Autodesk Fusion 360 part; units mm, degrees
(part 21 of 21)
  spline S194 degree 5 poles (-22.8173, 2.8931) (-22.8112, 2.8891) (-22.799, 2.8811) (-22.7807, 2.8692) (-22.7562, 2.8533) (-22.7256, 2.8337) (-22.695, 2.8142) (-22.6643, 2.7948) (-22.6336, 2.7755) (-22.6028, 2.7564) (-22.572, 2.7374) (-22.5411, 2.7186) (-22.5102, 2.6999) (-22.4793, 2.6814) (-22.4483, 2.6629) (-22.4173, 2.6447) (-22.3863, 2.6265) (-22.3552, 2.6085) (-22.3241, 2.5907) (-22.2929, 2.573) (-22.2617, 2.5554) (-22.2305, 2.538) (-22.1992, 2.5208) (-22.1679, 2.5037) (-22.1365, 2.4867) (-22.1051, 2.4699) (-22.0737, 2.4533) (-22.0422, 2.4368) (-22.0107, 2.4205) (-21.9792, 2.4043) (-21.9476, 2.3883) (-21.9159, 2.3724) (-21.8843, 2.3567) (-21.8526, 2.3412) (-21.8209, 2.3259) (-21.7891, 2.3107) (-21.7573, 2.2957) (-21.7254, 2.2808) (-21.6935, 2.2661) (-21.6616, 2.2517) (-21.6296, 2.2373) (-21.5976, 2.2232) (-21.5656, 2.2093) (-21.5335, 2.1955) (-21.5014, 2.1819) (-21.4693, 2.1686) (-21.4371, 2.1554) (-21.4048, 2.1424) (-21.3726, 2.1296) (-21.3403, 2.1171) (-21.3079, 2.1047) (-21.2755, 2.0926) (-21.2431, 2.0807) (-21.2107, 2.069) (-21.1782, 2.0575) (-21.1456, 2.0462) (-21.113, 2.0352) (-21.0804, 2.0245) (-21.0478, 2.0141) (-21.0151, 2.0039) (-20.9823, 1.9939) (-20.9495, 1.9842) (-20.9167, 1.9748) (-20.8838, 1.9657) (-20.8509, 1.9569) (-20.8179, 1.9485) (-20.7906, 1.9419) (-20.7698, 1.9371) (-20.7556, 1.9339) (-20.748, 1.9323) (-20.7471, 1.9321) knots -1 -1 -1 -1 -1 -1 -0.98571429 -0.97142857 -0.95714286 -0.94285714 -0.92857143 -0.91428571 -0.9 -0.88571429 -0.87142857 -0.85714286 -0.84285714 -0.82857143 -0.81428571 -0.8 -0.78571429 -0.77142857 -0.75714286 -0.74285714 -0.72857143 -0.71428571 -0.7 -0.68571429 -0.67142857 -0.65714286 -0.64285714 -0.62857143 -0.61428571 -0.6 -0.58571429 -0.57142857 -0.55714286 -0.54285714 -0.52857143 -0.51428571 -0.5 -0.48571429 -0.47142857 -0.45714286 -0.44285714 -0.42857143 -0.41428571 -0.4 -0.38571429 -0.37142857 -0.35714286 -0.34285714 -0.32857143 -0.31428571 -0.3 -0.28571429 -0.27142857 -0.25714286 -0.24285714 -0.22857143 -0.21428571 -0.2 -0.18571429 -0.17142857 -0.15714286 -0.14285714 -0.12857143 -0.11428571 -0.1 -0.08571429 -0.07142857 -0.06937658 -0.06937658 -0.06937658 -0.06937658 -0.06937658 -0.06937658
  spline S195 degree 3 poles (-20.6687, 1.8256) (-20.6676, 1.8385) (-20.669, 1.8516) (-20.6767, 1.8765) (-20.683, 1.888) (-20.6984, 1.9066) (-20.7068, 1.914) (-20.7258, 1.9255) (-20.7362, 1.9297) (-20.7471, 1.9321) knots 0 0 0 0 0.003906 0.003906 0.007813 0.007813 0.011148 0.011148 0.014483 0.014483 0.014483 0.014483
  circle A128 centre (0, 0) radius 7.5
  circle A129 centre (0, 0) radius 20
  line L20 (0, -30) -> (0, 28)
  dimension "d17" = 15
  dimension "d18" = 40
  constraint coincident A1.centre A3.centre
  constraint vertical L20
  measures "d17" diameter of A128
  measures "d18" diameter of A129
extrude "Estrusione3" cut sketch "Schizzo1 (3)" against normal blind 1 contours A128 A129 L20 picked at (7.7253, -13.7757) bodies 1 in component "Spur Gear (44 teeth)"
sketch "Schizzo2 (3)" plane through (0, 0, 2) normal (0, 0, 1) x (-1, 0, 0)
  line L0 (0, -7.5) -> (0, -20)
  arc A0 (0, -20) -> (0, 20) centre (0, 0) ccw
  line L1 (0, 20) -> (0, 7.5)
  arc A1 (0, -7.5) -> (0, 7.5) centre (0, 0) ccw
  line L2 (4.9545, 6.2187) -> (4.9545, -15.7813) construction
  line L3 (4.9545, -15.7813) -> (14.9545, -15.7813) construction
  line L4 (14.9545, -15.7813) -> (14.9545, 6.2187) construction
  line L5 (14.9545, 6.2187) -> (4.9545, 6.2187) construction
  dimension "d21" = 5
  text T0 "60m" font "Arial" height 5 bold align left top in box 22 x 10 at (4.9545, 6.2187) x (0, -1) y (1, 0) spacing 1 kerned
extrude "Estrusione4" add sketch "Schizzo2 (3)" along normal blind 1 text T0 bodies 1 in component "Spur Gear (44 teeth)"
component "Spur Gear (44 teeth)" placed x (1, 0, 0) y (0, 1, 0) z (0, 0, 1) at (0, 0, 0)
component "Spur Gear (10 teeth)" placed x (1, 0, 0) y (0, 1, 0) z (0, 0, 1) at (0, 0, 0)
